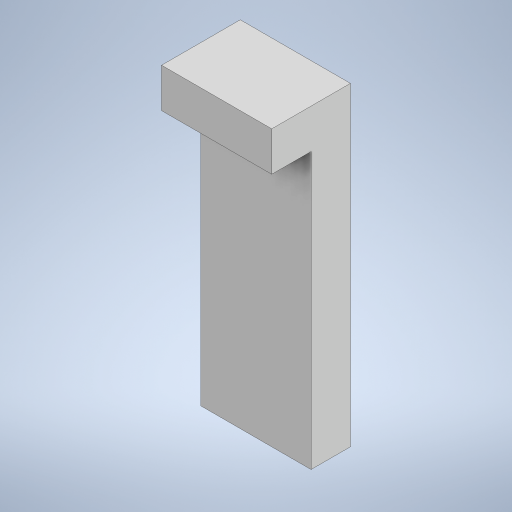
# Autodesk Inventor part: Pasador
Saved by Autodesk Inventor 2024 (Build 280153000, 153)
## iProperties
Created: 2024-03-06
Part Number: Pasador
Material: Genérico
Document SubType Name: Modeling
Designer: yovan
Density: 1 g/cm^3
Appearance: Valor por defecto
Author: yovan
Autodesk Inventor part; units mm, degrees
ref_plane "YZ Plane" through (0, 0, 0) normal (1, 0, 0) x (0, 1, 0)
ref_plane "XZ Plane" through (0, 0, 0) normal (0, 1, 0) x (-1, 0, 0)
ref_plane "XY Plane" through (0, 0, 0) normal (0, 0, 1) x (1, 0, 0)
sketch "Boceto1" plane through (0, 0, 0) normal (0, 0, 1) x (1, 0, 0)
  line L0 (0, 0) -> (14, 0)
  line L1 (14, 0) -> (14, 40)
  line L2 (14, 40) -> (0, 40)
  line L3 (0, 40) -> (0, 0)
  dimension "d0" = 14
  dimension "d1" = 40
  constraints: 8 end point, 2 parallel, 1 horizontal, 1 perpendicular
  measures "d0" distance of L2.end L1.end
  measures "d1" distance of L1.end L0.end
extrude "Extrusión1" add sketch "Boceto1" along normal blind 5
sketch "Boceto2" plane through (0, 0, 5) normal (0, 0, 1) x (1, 0, 0)
  line L0 (14, 40) -> (0, 40) projected
  line L1 (14, 40) -> (0, 40)
  line L2 (0, 40) -> (0, 35)
  line L3 (0, 35) -> (14, 35)
  line L4 (14, 35) -> (14, 40)
  point P0 (0, 0)
  dimension "d4" = 14
  dimension "d5" = 5
  constraints: 8 end point, 2 parallel, 1 horizontal, 1 perpendicular
  measures "d4" distance of L3.end L2.end
  measures "d5" distance of L2.end L1.end
extrude "Extrusión2" add sketch "Boceto2" along normal blind 5
